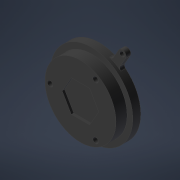
# Autodesk Inventor part: Planet Carrier 3
Saved by Autodesk Inventor 2021 (Build 250183000, 183)
## iProperties
Created: 2025-03-15
Part Number: Planet Carrier 3
Material: Generic
Document SubType Name: Modeling
Designer: rocke
Density: 0.448865 g/cm^3
Appearance: Default
Mass: 9.25 g
Surface Area: 65.8094 cm^2
Volume: 20.6075 cm^3
Author: rocke
Autodesk Inventor part; units mm, degrees
ref_plane "YZ Plane" through (0, 0, 0) normal (1, 0, 0) x (0, 1, 0)
ref_plane "XZ Plane" through (0, 0, 0) normal (0, 1, 0) x (-1, 0, 0)
sketch "Sketch1" plane through (0, 0, 0) normal (0, 0, 1) x (1, 0, 0)
  circle A0 centre (0, 0) radius 22.4
  dimension "d0" = 44.8
  constraints: 1 centre point, 1 coincident
  measures "d0" diameter of A0
extrude "Extrusion1" add sketch "Sketch1" along normal blind 7
sketch "Sketch2" plane through (0, 0, 0) normal (0, 0, -1) x (-1, 0, 0)
  circle A0 centre (0, 0) radius 26
  dimension "d3" = 52
  constraints: 1 centre point, 1 coincident
  measures "d3" diameter of A0
extrude "Extrusion2" add sketch "Sketch2" along normal blind 5
sketch "Sketch3" plane through (0, 0, -5) normal (0, 0, -1) x (-1, 0, 0)
  line L0 (22.23, 0) -> (20.6925, -2.663)
  line L1 (20.6925, -2.663) -> (17.6175, -2.663)
  line L2 (17.6175, -2.663) -> (16.08, 0)
  line L3 (16.08, 0) -> (17.6175, 2.663)
  line L4 (17.6175, 2.663) -> (20.6925, 2.663)
  line L5 (20.6925, 2.663) -> (22.23, 0)
  line L6 (-11.115, 19.2517) -> (-8.04, 19.2517)
  line L7 (-8.04, 19.2517) -> (-6.5025, 16.5887)
  line L8 (-6.5025, 16.5887) -> (-8.04, 13.9257)
  line L9 (-8.04, 13.9257) -> (-11.115, 13.9257)
  line L10 (-11.115, 13.9257) -> (-12.6525, 16.5887)
  line L11 (-12.6525, 16.5887) -> (-11.115, 19.2517)
  line L12 (-11.115, -19.2517) -> (-12.6525, -16.5887)
  line L13 (-12.6525, -16.5887) -> (-11.115, -13.9257)
  line L14 (-11.115, -13.9257) -> (-8.04, -13.9257)
  line L15 (-8.04, -13.9257) -> (-6.5025, -16.5887)
  line L16 (-6.5025, -16.5887) -> (-8.04, -19.2517)
  line L17 (-8.04, -19.2517) -> (-11.115, -19.2517)
  point P0 (0, 0)
  point P1 (19.155, 0)
  point P2 (-9.5775, 16.5887)
  point P3 (-9.5775, -16.5887)
  dimension "d6" = 3.075
  dimension "d7" = 19.155
  dimension "d10" = 360
  constraints: 36 end point, 53 other
  measures "d6" distance of L0.start point (19.155, 0)
  measures "d7" distance of point (19.155, 0) point (0, 0)
extrude "Extrusion3" cut sketch "Sketch3" against normal blind 4
sketch "Sketch4" plane through (0, 0, -5) normal (0, 0, -1) x (-1, 0, 0)
  circle A0 centre (19.155, 0) radius 1.75
  circle A1 centre (-9.5775, 16.5887) radius 1.75
  circle A2 centre (-9.5775, -16.5887) radius 1.75
  point P0 (0, 0)
  dimension "d14" = 3.5
  dimension "d15" = 19.155
  dimension "d18" = 360
  constraints: 3 centre point, 7 other
  measures "d14" diameter of A0
  measures "d15" distance of A0.centre point (0, 0)
extrude "Extrusion4" cut sketch "Sketch4" against normal through all
sketch "Sketch5" plane through (0, 0, 7) normal (0, 0, 1) x (1, 0, 0)
  line L0 (-11.547, 0) -> (-5.7735, 10)
  line L1 (-5.7735, 10) -> (5.7735, 10)
  line L2 (5.7735, 10) -> (11.547, 0)
  line L3 (11.547, 0) -> (5.7735, -10)
  line L4 (5.7735, -10) -> (-5.7735, -10)
  line L5 (-5.7735, -10) -> (-11.547, 0)
  point P0 (0, 0)
  point P1 (0, 0)
  dimension "d22" = 10
  constraints: 12 end point, 1 coincident, 1 horizontal, 13 other
  measures "d22" distance from line of L1 point (0, 0)
extrude "Extrusion5" cut sketch "Sketch5" against normal blind 1.5
ref_plane "Work Plane1" through (0, 0, 6.5) normal (0, 0, 1) x (1, 0, 0)
sketch "Sketch6" plane through (0, 0, 6.5) normal (0, 0, 1) x (1, 0, 0)
  circle A0 centre (0, 0) radius 22.5
  circle A1 centre (0, 0) radius 22.4 projected
  circle A2 centre (0, 0) radius 21.1
  dimension "d26" = 45
  dimension "d27" = 42.2
  constraints: 2 centre point, 2 coincident
  measures "d26" diameter of A0
  measures "d27" diameter of A2
extrude "Extrusion6" [suppressed]
sketch "Sketch7" plane through (0, 0, -5) normal (0, 0, -1) x (-1, 0, 0)
  point P0 (0, 0)
sketch "Sketch8" plane through (0, 0, -5) normal (0, 0, 1) x (1, 0, 0)
  line L0 (0, 0) -> (17.25, 29.8779)
  line L1 (0, 0) -> (34.5, 0) construction
  circle A0 centre (0, 0) radius 26 projected
  line L2 (13, 22.5167) -> (17.25, 29.8779) construction
  line L3 (15.1651, 21.2667) -> (19.4151, 28.6279)
  line L4 (15.0849, 31.1279) -> (10.8349, 23.7667)
  arc A1 (10.8349, 23.7667) -> (15.1651, 21.2667) centre (13, 22.5167) ccw
  arc A2 (19.4151, 28.6279) -> (15.0849, 31.1279) centre (17.25, 29.8779) ccw
  point P0 (15.125, 26.1973)
  point P1 (10.7773, 23.6611)
  point P2 (15.1025, 21.164)
  dimension "d30" = 34.5
  dimension "d31" = 60
  dimension "d32" = 5
  constraints: 12 end point, 4 point on circle, 4 tangent, 2 centre point, 1 collinear, 1 equal length, 1 horizontal, 1 midpoint, 1 parallel, 1 point on line, 2 other
  measures "d30" distance of L0.start L0.end
  measures "d31" angle of L1 L0
  measures "d32" diameter of A2
extrude "Extrusion7" add sketch "Sketch8" along normal blind 3 contours A0 A1 L4 A2 L3
sketch "Sketch9" plane through (0, 0, -2) normal (0, 0, 1) x (1, 0, 0)
  arc A0 (19.4151, 28.6279) -> (15.0849, 31.1279) centre (17.25, 29.8779) ccw projected
  circle A1 centre (17.25, 29.8779) radius 1.55
  point P0 (0, 0)
  dimension "d35" = 3.1
  constraints: 1 centre point, 1 coincident
  measures "d35" diameter of A1
extrude "Extrusion8" cut sketch "Sketch9" against normal blind 2
fillet "Fillet1" radius 2 2 edges at (15.1025, 21.164, -3.5) (10.7773, 23.6611, -3.5)
body "Solid1"
